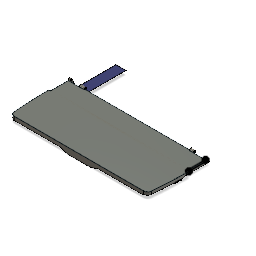
Psion Keyboard (Autodesk Fusion 360 design; units mm, degrees)
Autodesk Fusion 360 part; units mm, degrees
sketch "Sketch1" plane through (0, 0, 0) normal (0, 1, 0) x (1, 0, 0)
  line L0 (0, 0) -> (171.3, 0)
  line L1 (171.3, 0) -> (171.3, -71.5)
  line L2 (171.3, -71.5) -> (0, -71.5)
  line L3 (0, -71.5) -> (0, 0)
  line L4 (171.3, 0) -> (169.3, 0)
  line L5 (169.3, 0) -> (169.3, -23.3)
  line L6 (169.3, -23.3) -> (171.3, -23.3)
  line L7 (171.3, -23.3) -> (171.3, 0)
  line L8 (0, 0) -> (2, 0)
  line L9 (2, 0) -> (2, -23.3)
  line L10 (2, -23.3) -> (0, -23.3)
  line L11 (0, -23.3) -> (0, 0)
  arc A0 (0, -23.3) -> (2.4, -71.5) centre (485.2085, -23.3) ccw
  arc A1 (168.9, -71.5) -> (171.3, -23.3) centre (-313.9083, -23.3) ccw
  line L12 (2, 0) -> (0, 0)
  line L13 (0, 0) -> (0, -20.8)
  line L14 (0, -20.8) -> (2, -20.8)
  line L15 (2, -20.8) -> (2, 0)
  arc A2 (0, -23.3) -> (2, -20.8) centre (-0.5625, -20.8) ccw
  line L16 (171.3, 0) -> (169.3, 0)
  line L17 (169.3, 0) -> (169.3, -20.8)
  line L18 (169.3, -20.8) -> (171.3, -20.8)
  line L19 (171.3, -20.8) -> (171.3, 0)
  arc A3 (169.3, -20.8) -> (171.3, -23.3) centre (171.8625, -20.8) ccw
  dimension "d1" = 171.3
  dimension "d2" = 71.5
  dimension "d3" = 23.3
  dimension "d4" = 2
  dimension "d5" = 2
  dimension "d6" = 23.3
  dimension "d7" = 2.4
  dimension "d8" = 2.4
  dimension "d15" = 2.5
  dimension "d16" = 2.5
  constraint horizontal L0
  constraint vertical L1
  constraint horizontal L2
  constraint vertical L3
  constraint coincident L0.start L3.end
  constraint horizontal L4
  constraint vertical L5
  constraint horizontal L6
  constraint vertical L7
  constraint horizontal L8
  constraint vertical L9
  constraint horizontal L10
  constraint vertical L11
  constraint coincident L2 A0.end
  constraint tangent L11 A0
  constraint coincident L2 A1.start
  constraint tangent L7 A1
  constraint horizontal L12
  constraint vertical L13
  constraint horizontal L14
  constraint vertical L15
  constraint coincident L3 L13.end
  constraint tangent L15 A2
  constraint horizontal L16
  constraint vertical L17
  constraint horizontal L18
  constraint vertical L19
  constraint coincident L5 L17.end
  constraint tangent L17 A3
  measures "d1" distance of L1 L3
  measures "d2" distance of L0 L2
  measures "d3" distance of L4 L6
  measures "d4" distance of L1 L5
  measures "d5" distance of L3 L9
  measures "d6" distance of L0 L10
  measures "d7" horizontal distance of L2.end A0.end
  measures "d8" horizontal distance of L1.end A1.start
  measures "d15" distance of L10 L14
  measures "d16" distance of L6 L18
extrude "Extrude1" add sketch "Sketch1" along normal blind 4.7 contours L0 L2 L5 L6 L9 L10 A0 A1 L15 L17 | L9 L10 A2 | L5 L6 A3 makes body 1
sketch "Right Arm" plane through (169.3, 0, 0) normal (1, 0, 0) x (0, 0, -1)
  line L0 (-20.8, 0) -> (0, 0)
  line L1 (0, 0) -> (0, 4.7)
  line L2 (0, 4.7) -> (-20.8, 4.7)
  line L3 (-20.8, 4.7) -> (-20.8, 0)
  circle A0 centre (0.5, 5.2) radius 1.5
  line L4 (0, 0) -> (4.1, 0)
  line L5 (4.1, 0) -> (1.9006, 5.737)
  circle A1 centre (0.5, 5.2) radius 0.5
  dimension "d20" = 0.5
  dimension "d21" = 0.5
  dimension "d22" = 3
  dimension "d23" = 4.1
  dimension "d26" = 1
  constraint coincident L0.end L1.start
  constraint perpendicular L1 L4
  constraint tangent A0 L5
  constraint coincident A0 L5.end
  constraint concentric A0 A1
  measures "d20" horizontal distance of L1.end A0.centre
  measures "d21" vertical distance of L1.end A0.centre
  measures "d22" diameter of A0
  measures "d23" horizontal distance of L0.end L4.end
  measures "d26" diameter of A1
extrude "Extrude3" cut sketch "Right Arm" against normal blind 14.74 contours L1 L2 A0 | L1 L2 A0 bodies 1
extrude "Extrude2" add sketch "Right Arm" against normal blind 19.57 contours L1 L2 A0 | L1 L2 A0 bodies 1
extrude "Extrude4" cut sketch "Right Arm" against normal blind 14.74 contours L1 L2 A0 | L1 L2 A0 bodies 1
extrude "Extrude5" add sketch "Right Arm" against normal blind 2.24 contours L1 A0 L4 L5 | L1 L2 A0 | L1 L2 A0 bodies 1
sketch "Left Arm" plane through (2, 0, 0) normal (-1, 0, 0) x (0, 0, 1)
  line L0 (0, 0) -> (20.8, 0)
  line L1 (20.8, 0) -> (20.8, 4.7)
  line L2 (20.8, 4.7) -> (0, 4.7)
  line L3 (0, 4.7) -> (0, 0)
  circle A0 centre (-0.5, 5.2) radius 1.5
  line L4 (0, 0) -> (-4.1, 0)
  line L5 (-4.1, 0) -> (-1.766, 6.0881)
  circle A1 centre (-0.5, 5.2) radius 0.5
  dimension "d42" = 3
  dimension "d43" = 1
  dimension "d44" = 0.5
  dimension "d45" = 0.5
  dimension "d46" = 4.1
  constraint coincident L0.start L3.end
  constraint perpendicular L3 L4
  constraint concentric A0 A1
  constraint tangent A0 L5
  measures "d42" diameter of A0
  measures "d43" diameter of A1
  measures "d44" vertical distance of L2.end A0.centre
  measures "d45" horizontal distance of L2.end A0.centre
  measures "d46" horizontal distance of L0.start L4.end
extrude "Extrude6" add sketch "Left Arm" against normal blind 19.52 contours L2 L3 A0 | L2 L3 A0 bodies 1
extrude "Extrude7" cut sketch "Left Arm" against normal blind 13.64 contours L2 L3 A0 | L2 L3 A0 bodies 1
extrude "Extrude8" add sketch "Left Arm" against normal blind 2.24 contours L3 A0 L4 L5 | L2 L3 A0 | L2 L3 A0 bodies 1
sketch "Cable Cutaway" plane through (0, 0, 0) normal (0, 0, -1) x (-1, 0, 0)
  line L0 (-4.24, 0) -> (-4.24, 3.7858)
  line L1 (-4.24, 3.7858) -> (-15.64, 3.7858)
  line L2 (-15.64, 3.7858) -> (-21.52, 3.7858)
  line L3 (-21.52, 3.7858) -> (-21.52, 4.7)
  line L4 (-21.52, 4.7) -> (-149.73, 4.7)
  line L5 (-149.73, 4.7) -> (-149.73, 3.7858)
  line L6 (-149.73, 3.7858) -> (-154.56, 3.7858)
  line L7 (-154.56, 3.7858) -> (-167.06, 3.7858)
  line L8 (-167.06, 3.7858) -> (-167.06, 0)
  line L9 (-167.06, 0) -> (-4.24, 0)
  line L10 (-11.24, 0) -> (-30.82, 0)
  line L11 (-30.82, 0) -> (-30.82, 1.75)
  line L12 (-30.82, 1.75) -> (-11.24, 1.75)
  line L13 (-11.24, 1.75) -> (-11.24, 0)
  dimension "d53" = 7
  dimension "d57" = 19.58
  dimension "d59" = 1.75
  constraint horizontal L10
  constraint vertical L11
  constraint horizontal L12
  constraint vertical L13
  constraint coincident L9 L10.start
  measures "d53" horizontal distance of L0.start L10.start
  measures "d57" horizontal distance of L10.start L10.end
  measures "d59" vertical distance of L10.end L11.end
extrude "Extrude9" cut sketch "Cable Cutaway" against normal blind 2 contours L9 L10 L11 L12 L13 bodies 1
sketch "Cable Extrusion" plane through (0, 0, 2) normal (0, 0, -1) x (-1, 0, 0)
  line L0 (-11.24, 1.75) -> (-30.82, 1.75)
  line L1 (-30.82, 1.75) -> (-30.82, 0)
  line L2 (-30.82, 0) -> (-11.24, 0)
  line L3 (-11.24, 0) -> (-11.24, 1.75)
  line L4 (-11.24, 1.75) -> (-29.74, 1.75)
  line L5 (-29.74, 1.75) -> (-29.74, 1.62)
  line L6 (-29.74, 1.62) -> (-11.24, 1.62)
  line L7 (-11.24, 1.62) -> (-11.24, 1.75)
  dimension "d63" = 0.13
  dimension "d64" = 18.5
  constraint horizontal L4
  constraint vertical L5
  constraint horizontal L6
  constraint vertical L7
  constraint coincident L0.start L3.end
  measures "d63" distance of L4 L6
  measures "d64" horizontal distance of L5.end L6.end
extrude "Extrude10" add sketch "Cable Extrusion" along normal blind 50 separate body contours L0 L3 L4 L5 L6 L7 makes body 2
sketch "Cable" plane through (0, 1.62, 0) normal (0, -1, 0) x (1, 0, 0)
  line L0 (29.74, 2) -> (11.24, 2)
  line L1 (11.24, 2) -> (11.24, -48)
  line L2 (11.24, -48) -> (29.74, -48)
  line L3 (29.74, -48) -> (29.74, 2)
  line L4 (11.24, -48) -> (23.74, -48)
  line L5 (23.74, -48) -> (23.74, -3)
  line L6 (23.74, -3) -> (11.24, -3)
  line L7 (11.24, -3) -> (11.24, -48)
  line L8 (29.74, 2) -> (23.74, -3)
  dimension "d69" = 12.5
  dimension "d72" = 5
  constraint horizontal L4
  constraint vertical L5
  constraint horizontal L6
  constraint vertical L7
  constraint coincident L1.end L2.start
  constraint coincident L0.start L3.end
  measures "d69" distance of L5 L7
  measures "d72" distance of L0 L6
extrude "Extrude11" cut sketch "Cable" against normal blind 0.13 contours L0 L1 L6 L8 | L1 L2 L4 L5 L6 L7 keep common part bodies 2
sketch "Hooks" plane through (0, 0, 0) normal (0, -1, 0) x (1, 0, 0)
  line L0 (11.24, 0) -> (11.24, 2)
  line L1 (11.24, 2) -> (30.82, 2)
  line L2 (30.82, 2) -> (30.82, 0)
  line L3 (30.82, 0) -> (167.06, 0)
  line L4 (167.06, 0) -> (167.06, -4.1)
  line L5 (167.06, -4.1) -> (169.3, -4.1)
  line L6 (169.3, -4.1) -> (169.3, 20.8)
  arc A0 (171.3, 23.3) -> (169.3, 20.8) centre (171.8625, 20.8) ccw
  arc A1 (171.3, 23.3) -> (168.9, 71.5) centre (-313.9083, 23.3) ccw
  line L7 (168.9, 71.5) -> (2.4, 71.5)
  arc A2 (2.4, 71.5) -> (0, 23.3) centre (485.2085, 23.3) ccw
  arc A3 (2, 20.8) -> (0, 23.3) centre (-0.5625, 20.8) ccw
  line L8 (2, 20.8) -> (2, -4.1)
  line L9 (2, -4.1) -> (4.24, -4.1)
  line L10 (4.24, -4.1) -> (4.24, 0)
  line L11 (4.24, 0) -> (11.24, 0)
  line L12 (2, -4.1) -> (169.3, -4.1)
  line L13 (169.3, -4.1) -> (169.3, 38.4)
  line L14 (169.3, 38.4) -> (2, 38.4)
  line L15 (2, 38.4) -> (2, -4.1)
  line L16 (169.3, 20.8) -> (169.3, 0)
  line L17 (163.3, 38.4) -> (5, 38.4)
  line L18 (5, 38.4) -> (5, 71.5)
  line L19 (5, 71.5) -> (163.3, 71.5)
  line L20 (163.3, 71.5) -> (163.3, 38.4)
  line L21 (169.3, 38.4) -> (163.3, 38.4)
  line L22 (163.3, 38.4) -> (163.3, 30.26)
  line L23 (163.3, 30.26) -> (169.3, 30.26)
  line L24 (169.3, 30.26) -> (169.3, 38.4)
  line L25 (163.3, 30.26) -> (161.7, 30.26)
  line L26 (161.7, 30.26) -> (161.7, 38.4)
  line L27 (161.7, 38.4) -> (163.3, 38.4)
  line L28 (163.3, 38.4) -> (163.3, 30.26)
  line L29 (2, 38.4) -> (5, 38.4)
  line L30 (5, 38.4) -> (5, 30.26)
  line L31 (5, 30.26) -> (2, 30.26)
  line L32 (2, 30.26) -> (2, 38.4)
  line L33 (5, 30.26) -> (6.6, 30.26)
  line L34 (6.6, 30.26) -> (6.6, 38.4)
  line L35 (6.6, 38.4) -> (5, 38.4)
  line L36 (5, 38.4) -> (5, 30.26)
  dimension "d75" = 42.5
  dimension "d89" = 1.6
  dimension "d90" = 1.6
  dimension "d91" = 8.14
  dimension "d92" = 8.14
  dimension "d156" = 3
  dimension "d157" = 6
  constraint horizontal L12
  constraint vertical L13
  constraint horizontal L14
  constraint vertical L15
  constraint coincident L8.end L9.start
  constraint collinear L13 L16
  constraint horizontal L17
  constraint vertical L18
  constraint horizontal L19
  constraint vertical L20
  constraint collinear L14 L17
  constraint horizontal L21
  constraint vertical L22
  constraint horizontal L23
  constraint vertical L24
  constraint horizontal L25
  constraint vertical L26
  constraint horizontal L27
  constraint vertical L28
  constraint coincident L14 L26.end
  constraint horizontal L29
  constraint vertical L30
  constraint horizontal L31
  constraint vertical L32
  constraint horizontal L33
  constraint vertical L34
  constraint horizontal L35
  constraint vertical L36
  constraint coincident L17 L34.end
  constraint collinear L20 L28
  constraint collinear L18 L36
  measures "d75" distance of L12 L14
  measures "d89" distance of L26 L28
  measures "d90" distance of L34 L36
  measures "d91" distance of L29 L31
  measures "d92" distance of L21 L23
  measures "d156" horizontal distance of L30.end L31.end
  measures "d157" horizontal distance of L22.end L23.end
extrude "Extrude17" add sketch "Hooks" along normal blind 2 contours L13 L14 L21 L22 L23 L24 L28 | L14 L17 L22 L25 L26 L27 L28 bodies 1
extrude "Extrude16" add sketch "Hooks" along normal blind 2 contours L13 L14 L21 L22 L23 L24 L28 | L14 L17 L22 L25 L26 L27 L28 bodies 1
extrude "Extrude15" add sketch "Hooks" along normal blind 2 contours L13 L14 L21 L22 L23 L24 L28 | L14 L17 L22 L25 L26 L27 L28 bodies 1
extrude "Extrude14" add sketch "Hooks" along normal blind 1 contours L14 L17 L22 L25 L26 L27 L28 bodies 1
extrude "Extrude13" add sketch "Hooks" along normal blind 2 contours L13 L14 L21 L22 L23 L24 L28 | L14 L17 L22 L25 L26 L27 L28 bodies 1
extrude "Extrude12" cut sketch "Hooks" against normal blind 1 contours L7 A2 A3 L14 L15 L18 L29 L32 | A0 A1 L7 L13 L14 L20 L21 L24 bodies 1
fillet "Fillet1" radius 5 1 edges at (2.4, 2.85, 71.5) on bodies 1
fillet "Fillet2" radius 5 1 edges at (168.9, 2.85, 71.5) on bodies 1
sketch "Right Hook Inset" plane through (161.7, 0, 0) normal (-1, 0, 0) x (0, 0, 1)
  line L0 (30.26, 0) -> (30.26, -2)
  line L1 (30.26, -2) -> (38.4, -2)
  line L2 (38.4, -2) -> (38.4, 0)
  line L3 (38.4, 0) -> (30.26, 0)
  line L4 (30.26, 0) -> (38.4, 0)
  line L5 (38.4, 0) -> (38.4, -1)
  line L6 (38.4, -1) -> (30.26, -1)
  line L7 (30.26, -1) -> (30.26, 0)
  line L8 (30.26, 0) -> (38.4, 0)
  dimension "d103" = 1
  constraint horizontal L4
  constraint vertical L5
  constraint horizontal L6
  constraint vertical L7
  constraint coincident L2 L5.end
  constraint coincident L0.start L3.end
  measures "d103" distance of L6 L8
extrude "Extrude18" cut sketch "Right Hook Inset" against normal blind 1.6 contours L0 L2 L3 L4 L5 L6 L7 L8 bodies 1
extrude "Extrude19" add sketch "Hooks" along normal blind 2 contours L14 L15 L29 L30 L31 L32 L36 | L14 L17 L30 L33 L34 L35 L36 bodies 1
sketch "Left Hook Inset" plane through (6.6, 0, 0) normal (1, 0, 0) x (0, 0, -1)
  line L0 (-30.26, 0) -> (-38.4, 0)
  line L1 (-38.4, 0) -> (-38.4, -2)
  line L2 (-38.4, -2) -> (-30.26, -2)
  line L3 (-30.26, -2) -> (-30.26, 0)
  line L4 (-38.4, 0) -> (-30.26, 0)
  line L5 (-30.26, 0) -> (-30.26, -1)
  line L6 (-30.26, -1) -> (-38.4, -1)
  line L7 (-38.4, -1) -> (-38.4, 0)
  line L8 (-30.26, 0) -> (-38.4, 0)
  dimension "d108" = 1
  constraint horizontal L4
  constraint vertical L5
  constraint horizontal L6
  constraint vertical L7
  constraint coincident L3 L5.end
  constraint coincident L0.end L1.start
  measures "d108" distance of L6 L8
extrude "Extrude20" cut sketch "Left Hook Inset" against normal blind 1.6 contours L0 L1 L3 L4 L5 L6 L7 L8 bodies 1
sketch "Front Feature" plane through (0, 0, 71.5) normal (0, 0, 1) x (1, 0, 0)
  line L0 (164.3529, 1) -> (164.3529, 4.7)
  line L1 (164.3529, 4.7) -> (6.9471, 4.7)
  line L2 (6.9471, 4.7) -> (6.9471, 0)
  line L3 (6.9471, 0) -> (163.3, 0)
  line L4 (63.15, 4.7) -> (108.15, 4.7)
  line L5 (108.15, 4.7) -> (108.15, -3)
  line L6 (108.15, -3) -> (63.15, -3)
  line L7 (63.15, -3) -> (63.15, 4.7)
  line L8 (75.1236, 0) -> (95.1236, 0)
  line L9 (95.1236, 0) -> (95.1236, -3)
  line L10 (95.1236, -3) -> (75.1236, -3)
  line L11 (75.1236, -3) -> (75.1236, 0)
  arc A0 (63.15, 0) -> (75.1236, -3) centre (75.1236, 22.3943) ccw
  arc A1 (95.1236, -3) -> (108.15, 0) centre (95.1236, 26.7814) ccw
  line L12 (163.3, 1) -> (164.3529, 1)
  line L13 (163.3, 0) -> (163.3, 1)
  dimension "d111" = 45
  dimension "d115" = 7.7
  dimension "d116" = 20
  constraint horizontal L4
  constraint vertical L5
  constraint horizontal L6
  constraint vertical L7
  constraint midpoint L1 L4
  constraint horizontal L8
  constraint vertical L9
  constraint horizontal L10
  constraint vertical L11
  constraint midpoint L3 L8
  constraint collinear L6 L10
  constraint coincident L7 A0.start
  constraint coincident L3 A0.start
  constraint tangent L10 A0
  constraint coincident L5 A1.end
  constraint coincident L3 A1.end
  constraint tangent L10 A1
  measures "d111" distance of L5 L7
  measures "d115" distance of L4 L6
  measures "d116" distance of L9 L11
extrude "Extrude21" add sketch "Front Feature" against normal blind 1 contours L3 L9 A1 | L3 L11 A0 | L3 L6 L8 L9 L10 L11 bodies 1
sketch "Front Hook" plane through (0, 0, 0) normal (0, -1, 0) x (1, 0, 0)
  line L0 (63.15, 70.5) -> (63.15, 71.5)
  line L1 (63.15, 71.5) -> (6.9471, 71.5)
  line L2 (5, 71.1053) -> (5, 38.4)
  line L3 (5, 38.4) -> (5, 30.26)
  line L4 (5, 30.26) -> (2, 30.26)
  line L5 (2, 30.26) -> (2, -4.1)
  line L6 (2, -4.1) -> (4.24, -4.1)
  line L7 (4.24, -4.1) -> (4.24, 0)
  line L8 (4.24, 0) -> (11.24, 0)
  line L9 (11.24, 0) -> (11.24, 2)
  line L10 (11.24, 2) -> (30.82, 2)
  line L11 (30.82, 2) -> (30.82, 0)
  line L12 (30.82, 0) -> (167.06, 0)
  line L13 (167.06, 0) -> (167.06, -4.1)
  line L14 (167.06, -4.1) -> (169.3, -4.1)
  line L15 (169.3, -4.1) -> (169.3, 30.26)
  line L16 (169.3, 30.26) -> (163.3, 30.26)
  line L17 (163.3, 30.26) -> (163.3, 38.4)
  line L18 (163.3, 38.4) -> (163.3, 71.5)
  line L19 (108.15, 71.5) -> (108.15, 70.5)
  line L20 (108.15, 70.5) -> (63.15, 70.5)
  line L21 (75.65, 70.5) -> (81.37, 70.5)
  line L22 (81.37, 70.5) -> (81.37, 66.2)
  line L23 (81.37, 66.2) -> (75.65, 66.2)
  line L24 (75.65, 66.2) -> (75.65, 70.5)
  arc A0 (6.9471, 71.5) -> (5, 71.1053) centre (6.9471, 66.5) ccw
  line L25 (163.3, 71.5) -> (108.15, 71.5)
  dimension "d123" = 12.5
  dimension "d124" = 5.72
  dimension "d125" = 4.3
  constraint horizontal L21
  constraint vertical L22
  constraint horizontal L23
  constraint vertical L24
  constraint coincident L20 L21.start
  measures "d123" distance of L0.start L24
  measures "d124" distance of L22 L24
  measures "d125" distance of L21 L23
extrude "Extrude22" add sketch "Front Hook" along normal blind 2 contours L20 L21 L22 L23 L24 bodies 1
sketch "Front Hook Right Inset" plane through (81.37, 0, 0) normal (1, 0, 0) x (0, 0, -1)
  line L0 (-66.2, 0) -> (-70.5, 0)
  line L1 (-70.5, 0) -> (-70.5, -2)
  line L2 (-70.5, -2) -> (-66.2, -2)
  line L3 (-66.2, -2) -> (-66.2, 0)
  line L4 (-66.2, 0) -> (-70.5, 0)
  line L5 (-70.5, 0) -> (-70.5, -1)
  line L6 (-70.5, -1) -> (-66.2, -1)
  line L7 (-66.2, -1) -> (-66.2, 0)
  dimension "d128" = 1
  constraint horizontal L4
  constraint vertical L5
  constraint horizontal L6
  constraint vertical L7
  constraint coincident L1 L5.end
  constraint coincident L0.start L3.end
  measures "d128" distance of L4 L6
extrude "Extrude23" cut sketch "Front Hook Right Inset" against normal blind 2.5 contours L0 L1 L3 L4 L5 L6 L7 bodies 1
sketch "Front Hook Left Inset" plane through (75.65, 0, 0) normal (-1, 0, 0) x (0, 0, 1)
  line L0 (70.5, 0) -> (66.2, 0)
  line L1 (66.2, 0) -> (66.2, -2)
  line L2 (66.2, -2) -> (70.5, -2)
  line L3 (70.5, -2) -> (70.5, 0)
  line L4 (66.2, 0) -> (70.5, 0)
  line L5 (70.5, 0) -> (70.5, -1)
  line L6 (70.5, -1) -> (66.2, -1)
  line L7 (66.2, -1) -> (66.2, 0)
  dimension "d132" = 1
  constraint horizontal L4
  constraint vertical L5
  constraint horizontal L6
  constraint vertical L7
  constraint coincident L3 L5.end
  constraint coincident L0.end L1.start
  measures "d132" distance of L4 L6
extrude "Extrude24" cut sketch "Front Hook Left Inset" against normal blind 2.5 contours L0 L1 L3 L4 L5 L6 L7 bodies 1
sketch "Left Side Detail Angle" plane through (2, 0, 0) normal (-1, 0, 0) x (0, 0, 1)
  circle A0 centre (-0.5, 5.2) radius 0.5
  line L0 (38.4, -2) -> (38.4, 1)
  line L1 (38.4, 1) -> (20.8, 1)
  line L2 (20.8, 1) -> (20.8, 4.7)
  line L3 (20.8, 4.7) -> (0.9142, 4.7)
  arc A1 (0.9142, 4.7) -> (-1.9006, 5.7369) centre (-0.5, 5.2) ccw
  line L4 (-1.9006, 5.7369) -> (-4.1, 0)
  line L5 (-4.1, 0) -> (30.26, 0)
  line L6 (30.26, 0) -> (30.26, -2)
  line L7 (30.26, -2) -> (38.4, -2)
  line L8 (20.8, 4.7) -> (26.8, 1)
  dimension "d141" = 6
  constraint coincident L2.end L3.start
  constraint coincident L1 L8.end
  measures "d141" horizontal distance of L1.end L8.end
sketch "Left Side Detail" plane through (0, 4.7, 0) normal (0, 1, 0) x (-1, 0, 0)
  arc A0 (-164.3529, 71.5) -> (-169.3326, 66.9498) centre (-164.3529, 66.5) ccw
  arc A1 (-169.3326, 66.9498) -> (-171.3, 23.3) centre (313.9083, 23.3) ccw
  arc A2 (-169.3, 20.8) -> (-171.3, 23.3) centre (-171.8625, 20.8) ccw
  line L0 (-169.3, 20.8) -> (-169.3, 0.9142)
  line L1 (-169.3, 0.9142) -> (-167.06, 0.9142)
  line L2 (-167.06, 0.9142) -> (-154.56, 0.9142)
  line L3 (-154.56, 0.9142) -> (-149.73, 0.9142)
  line L4 (-149.73, 0.9142) -> (-149.73, 0)
  line L5 (-149.73, 0) -> (-21.52, 0)
  line L6 (-21.52, 0) -> (-21.52, 0.9142)
  line L7 (-21.52, 0.9142) -> (-15.64, 0.9142)
  line L8 (-15.64, 0.9142) -> (-4.24, 0.9142)
  line L9 (-4.24, 0.9142) -> (-2, 0.9142)
  line L10 (-2, 0.9142) -> (-2, 20.8)
  arc A3 (0, 23.3) -> (-2, 20.8) centre (0.5625, 20.8) ccw
  arc A4 (0, 23.3) -> (-1.9674, 66.9498) centre (-485.2085, 23.3) ccw
  arc A5 (-1.9674, 66.9498) -> (-6.9471, 71.5) centre (-6.9471, 66.5) ccw
  line L11 (-6.9471, 71.5) -> (-164.3529, 71.5)
  line L12 (-2, 0.9142) -> (0, 0.9142)
  line L13 (0, 0.9142) -> (0, 23.3)
  line L14 (0, 23.3) -> (-2, 23.3)
  line L15 (-2, 23.3) -> (-2, 0.9142)
  constraint horizontal L12
  constraint vertical L13
  constraint horizontal L14
  constraint vertical L15
  constraint coincident A3.start A4.start
  constraint coincident L9.end L10.start
sweep "Sweep2" cut profiles "Left Side Detail" path "Left Side Detail Angle" along L8 section 1 contours L10 A3 L12 L13 L15 bodies 1
sketch "Right Side Detail Angle" plane through (169.3, 0, 0) normal (1, 0, 0) x (0, 0, -1)
  circle A0 centre (0.5, 5.2) radius 0.5
  line L0 (-38.4, 1) -> (-38.4, -2)
  line L1 (-38.4, -2) -> (-30.26, -2)
  line L2 (-30.26, -2) -> (-30.26, 0)
  line L3 (-30.26, 0) -> (4.1, 0)
  line L4 (4.1, 0) -> (1.9006, 5.737)
  arc A1 (1.9006, 5.737) -> (-0.9142, 4.7) centre (0.5, 5.2) ccw
  line L5 (-0.9142, 4.7) -> (-20.8, 4.7)
  line L6 (-20.8, 4.7) -> (-20.8, 1)
  line L7 (-20.8, 1) -> (-38.4, 1)
  line L8 (-20.8, 4.7) -> (-26.8, 1)
  dimension "d149" = 6
  constraint coincident L5.end L6.start
  constraint coincident L7 L8.end
  measures "d149" horizontal distance of L6.end L8.end
sketch "Right Side Detail" plane through (0, 4.7, 0) normal (0, 1, 0) x (-1, 0, 0)
  arc A0 (-164.3529, 71.5) -> (-169.3326, 66.9498) centre (-164.3529, 66.5) ccw
  arc A1 (-169.3326, 66.9498) -> (-171.3, 23.3) centre (313.9083, 23.3) ccw
  arc A2 (-169.3, 20.8) -> (-171.3, 23.3) centre (-171.8625, 20.8) ccw
  line L0 (-169.3, 20.8) -> (-169.3, 0.9142)
  line L1 (-169.3, 0.9142) -> (-167.06, 0.9142)
  line L2 (-167.06, 0.9142) -> (-154.56, 0.9142)
  line L3 (-154.56, 0.9142) -> (-149.73, 0.9142)
  line L4 (-149.73, 0.9142) -> (-149.73, 0)
  line L5 (-149.73, 0) -> (-21.52, 0)
  line L6 (-21.52, 0) -> (-21.52, 0.9142)
  line L7 (-21.52, 0.9142) -> (-15.64, 0.9142)
  line L8 (-15.64, 0.9142) -> (-4.24, 0.9142)
  line L9 (-4.24, 0.9142) -> (-2, 0.9142)
  line L10 (-2, 0.9142) -> (-2, 20.8)
  arc A3 (0, 23.3) -> (-2, 20.8) centre (0.5625, 20.8) ccw
  arc A4 (0, 23.3) -> (-1.9674, 66.9498) centre (-485.2085, 23.3) ccw
  arc A5 (-1.9674, 66.9498) -> (-6.9471, 71.5) centre (-6.9471, 66.5) ccw
  line L11 (-6.9471, 71.5) -> (-164.3529, 71.5)
  line L12 (-169.3, 0.9142) -> (-171.3, 0.9142)
  line L13 (-171.3, 0.9142) -> (-171.3, 23.3)
  line L14 (-171.3, 23.3) -> (-169.3, 23.3)
  line L15 (-169.3, 23.3) -> (-169.3, 0.9142)
  constraint horizontal L12
  constraint vertical L13
  constraint horizontal L14
  constraint vertical L15
  constraint coincident A1.end A2.end
  constraint coincident L0.end L1.start
sweep "Sweep3" cut profiles "Right Side Detail" path "Right Side Detail Angle" along L8 section 1 contours A2 L0 L12 L13 L15 bodies 1
equation "d1 = width"
equation "d2 = depth"
equation "d3 = depth - curveDepth"
equation "d4 = slideInset"
equation "d5 = slideInset"
equation "d6 = depth - curveDepth"
equation "d7 = curveInset"
equation "d8 = curveInset"
equation "depth = 71.5 mm"
equation "curveDepth = 48.2 mm"
equation "curveInset = 2.4 mm"
equation "slideInset = 2 mm"
equation "width = 171.3 mm"
equation "height = 4.7 mm"
equation "d15 = backCurveDepth"
equation "d16 = backCurveDepth"
equation "backCurveDepth = 2.5 mm"
equation "d18 = height"
equation "d20 = hingeOffset"
equation "d21 = hingeOffset"
equation "d22 = hingeDiameter"
equation "d23 = armDepth"
equation "hingeDiameter = 3 mm"
equation "armDepth = 4.1 mm"
equation "d26 = hingeDiameterInner"
equation "hingeDiameterInner = 1 mm"
equation "leftHingeEndWidth = 5.88 mm"
equation "rightHingeEndWidth = 4.83 mm"
equation "armWidth = 2.24 mm"
equation "leftHingeSlotWidth = 11.4 mm"
equation "rightHingeSlotWidth = 12.5 mm"
equation "d33 = -rightHingeEndWidth - rightHingeSlotWidth - armWidth"
equation "d35 = -rightHingeSlotWidth - armWidth"
equation "d37 = -rightHingeSlotWidth - armWidth"
equation "d39 = -armWidth"
equation "hingeOffset = 0.5 mm"
equation "d42 = hingeDiameter"
equation "d43 = hingeDiameterInner"
equation "d44 = hingeOffset"
equation "d45 = hingeOffset"
equation "d46 = armDepth"
equation "d47 = -leftHingeEndWidth - leftHingeSlotWidth - armWidth"
equation "d49 = -armWidth - leftHingeSlotWidth"
equation "d51 = -armWidth"
equation "d53 = cableCutoutRightOffset"
equation "cableCutoutRightOffset = 7 mm"
equation "cableCutoutWidth = 19.58 mm"
equation "cableCutoutDepth = 2 mm"
equation "d57 = cableCutoutWidth"
equation "cableCutoutHeight = 1.75 mm"
equation "d59 = cableCutoutHeight"
equation "d60 = -cableCutoutDepth"
equation "cableHeight = 0.13 mm"
equation "d63 = cableHeight"
equation "d64 = cableMaxWidth"
equation "cableMaxWidth = 18.5 mm"
equation "d66 = cableDepth"
equation "cableDepth = 50 mm"
equation "d69 = cableMinWidth"
equation "cableMinWidth = 12.5 mm"
equation "cableTransitionDepth = 5 mm"
equation "d72 = cableTransitionDepth"
equation "d73 = -cableHeight"
equation "d75 = sliderBackDepth"
equation "slideWidth = 158 mm"
equation "slideHeight = 1 mm"
equation "d79 = -slideHeight"
equation "sliderBackDepth = 42.5 mm"
equation "frontRadius = 5 mm"
equation "d83 = frontRadius"
equation "d84 = frontRadius"
equation "hookDepth = 8.14 mm"
equation "hookHeight = 2 mm"
equation "hookSpaceHeight = 1 mm"
equation "hookInset = 1.60 mm"
equation "d89 = hookInset"
equation "d90 = hookInset"
equation "d91 = hookDepth"
equation "d92 = hookDepth"
equation "d93 = hookHeight"
equation "d95 = hookSpaceHeight"
equation "d97 = hookHeight"
equation "d99 = hookHeight"
equation "d101 = hookHeight"
equation "d103 = hookSpaceHeight"
equation "d104 = -hookInset"
equation "d106 = hookHeight"
equation "d108 = hookSpaceHeight"
equation "d109 = -hookInset"
equation "d111 = frontFeatureWidth"
equation "frontFeatureWidth = 45 mm"
equation "frontFeatureDepth = 1 mm"
equation "frontFeatureHeight = 7.7 mm"
equation "d115 = frontFeatureHeight"
equation "d116 = frontFeatureInnerWidth"
equation "frontFeatureInnerWidth = 20 mm"
equation "d118 = -frontFeatureDepth"
equation "frontHookWidth = 5.72 mm"
equation "frontHookDepth = 4.3 mm"
equation "frontHookLeftOffset = 12.5 mm"
equation "d123 = frontHookLeftOffset"
equation "d124 = frontHookWidth"
equation "d125 = frontHookDepth"
equation "d126 = hookHeight"
equation "d128 = hookSpaceHeight"
equation "frontHookInsetWidth = 2.5 mm"
equation "d130 = -frontHookInsetWidth"
equation "d132 = hookSpaceHeight"
equation "d133 = -frontHookInsetWidth"
equation "d141 = sideDetailDepth"
equation "sideDetailDepth = 6 mm"
equation "d149 = sideDetailDepth"
equation "d156 = leftSlideMargin"
equation "d157 = rightSlideMargin"
equation "rightSlideMargin = 6 mm"
equation "leftSlideMargin = 3 mm"
named bodies: "Keyboard", "Cable"
